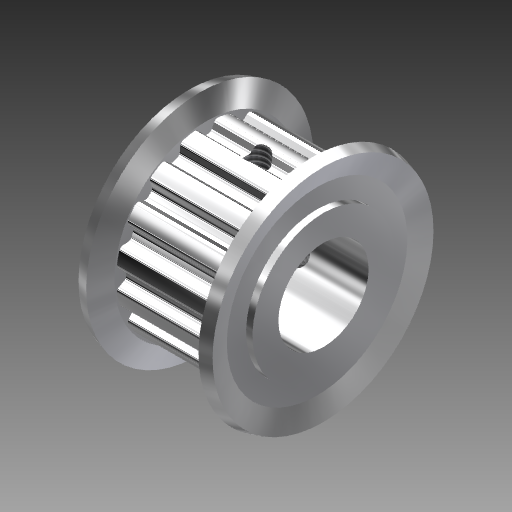
# Autodesk Inventor part: ATP16XL050-A-PUF_a
Saved by Autodesk Inventor 2019 (Build 230136000, 136)
## iProperties
Category: PARTsolutions
Company: MISUMI
Created: 2018-08-04
Part Number: ATP16XL050-A-PUF_a
Material: Aluminum 6061
Catalog Web Link: www.cadenas.de
Description: ATP_ _XL025, ATP_ _XL031, ATP_ _ XL037, ATP_ _XL050, BTP_ _XL025, BTP_ _XL031, BTP_ _XL037, BTP_ _XL050, KTP_ _XL025, KTP_ _XL031, KTP_ _ XL037, KTP_ _XL050, NTP_ _XL025, NTP_ _XL031, NTP_ _ XL037, NTP_ _XL050, MTP_ _XL025, MTP_ _ XL037, MTP_ _XL050, MTPB_ _XL025, MTPB_ _ XL037, MTPB_ _XL050, MTPP_ _XL025, MTPP_ _ XL037, MTPP_ _XL050, STP_ _XL025, STP_ _ XL037, STP_ _XL050_aI-Timing Pulleys XL Type
Vendor: MISUMI
Document SubType Name: Modeling
Designer: psadmin
Manufacturer: MISUMI
Mass: 19.1099 g
Surface Area: 46.6656 cm^2
Volume: 7.07773 cm^3
Density: 2.7 g/cm^3
Appearance: Aluminum - Flat
PSOL_IDENT_0: {$CADENAS_DATA\23d-libs\misumi\metric\51_timing_pulleys\timing_pulleys_inch\atp_xl_inch.prj},698 {VT
PSOL_IDENT_1: YP=3D},{NB=ATP16XL050-A-PUF_a},{LINA=ATP16XL050-A-PUF_a},{NN=ATP_ _XL025, ATP_ _XL031, ATP_ _ XL037,
PSOL_IDENT_2: ATP_ _XL050, BTP_ _XL025, BTP_ _XL031, BTP_ _XL037, BTP_ _XL050, KTP_ _XL025, KTP_ _XL031, KTP_ _ X
PSOL_IDENT_3: L037, KTP_ _XL050, NTP_ _XL025, NTP_ _XL031, NTP_ _ XL037, NTP_ _XL050, MTP_ _XL025, MTP_ _ XL037, M
PSOL_IDENT_4: TP_ _XL050, MTPB_ _XL025, MTPB_ _ XL037, MTPB_ _XL050, MTPP_ _XL025, MTPP_ _ XL037, MTPP_ _XL050, ST
PSOL_IDENT_5: P_ _XL025, STP_ _ XL037, STP_ _XL050_aI},{DATE=30.03.2018 07:26:26},{GEOMDATE=12.01.2011 12:59:00},{
PSOL_IDENT_6: VERSION=},{LINEID=30},{WBVAR=MATP,ST,TNW,PS,SHS,DD,ALT2,M,QSC,QFC,QTC,ALT7,K,KSC,KFC,KTC,ALT1,ALT3,A
PSOL_IDENT_7: LT4,ALT5,FC,ALT6,TPC,ALT8,BC,ALT9,SLH},{WBNUMERIC=DD,QSC,QFC,QTC,K,KSC,KFC,KTC,FC,TPC,BC,SLH}  {NB=A
PSOL_IDENT_8: TP16XL050-A-PUF_a},{LINA=ATP16XL050-A-PUF_a},{KT=DUMMY},{PN=ATP16XL050-A-PUF},{TYPE=ATP},{MATP=ATP},
PSOL_IDENT_9: {MATPA='ATP','2017 Aluminum Alloy (Duralumin)','MTP','1045 Carbon Steel','STP','304 Stainless Steel'
PSOL_IDENT_10: },{MATF=5052 Aluminum Alloy},{ST=CA},{HARD=-},{STA= 'CA' , 'Clear Anodize' , 'BA','Black Anodize','H
PSOL_IDENT_11: AT','Hard Clear Anodize','ENP' , 'Electroless Nickel Plating' },{NT=16},{TNW=XL050},{TNW1=      'XL0
PSOL_IDENT_12: 25','XL031','XL037','XL050'                            },{BW=12.7mm (1/2inch)},{A=14.0},{W=19.0},{L=
PSOL_IDENT_13: 28},{PS=A},{PSA='A','B'},{SHS=P},{SHS1= 'H','Inch Round Hole', 'P','Inch Round Hole + Tap','N','Inch
PSOL_IDENT_14: ANSI Key Groove Hole'},{SHS2=-PUF},{SHSA= 'H','Inch Round Hole', 'P','Inch Round Hole + Tap','N','I
PSOL_IDENT_15: nch ANSI Key Groove Hole'},{SHSB= 'H','Inch Round Hole', 'P','Inch Round Hole + Tap','N','Inch ANSI
PSOL_IDENT_16: Key Groove Hole'},{DD=0.5},{DDINCH=12.7},{DD1=0.25,0.3125,0.3750,0.5},{DDH=0.25,0.3125,0.3750,0.5},{
PSOL_IDENT_17: DDP=0.25,0.3125,0.3750,0.5},{DDN=0.3125,0.3750,0.5},{DDNK=10},{DDC=10,12},{DDV=5,6,6.35,7,8,9,10,11}
PSOL_IDENT_18: ,{DDF=5,6,6.35,7,8,9,10},{DDY=5,6,7,8,9,10,11,12},{DD635=13},{Z=0},{Z1=0},{ZQRMIN=15},{ZMAX=13},{ZA=
PSOL_IDENT_19: 0},{ZB=0},{ZAB=},{J=0},{JA=0},{JMAX=17.0},{JAB=},{QRMAX=14},{Q=0},{Q1=0},{Q2=},{R=0},{R1=0},{R2=},{S=
PSOL_IDENT_20: 0},{S1=0},{S2=},{SMAX=8},{T=0},{T1=0},{T2=},{TMAX=8},{PD=25.87},{OD=25.36},{D=0},{DB=17},{F=32},{E=2
PSOL_IDENT_21: 0},{DE=20},{BJS9=0},{TTTI=0},{TTT=0},{AC=-},{NDM=4.000},{WL=19},{ALT2=},{ALT2A='','N/A'},{QMIN=20},{
PSOL_IDENT_22: QMAX=13},{M=-},{MA= '-' },{MAA=},{NDMALT=0.000},{QSC=0},{QSCA=0},{QSCAA=},{QFC=0},{QFCA=0},{QFCAA=},
PSOL_IDENT_23: {QTC=0},{QTCA=0},{QTCAA=},{QCMIN=17},{QCMAX=16},{QC=0},{ALT7=},{ALT7A='','N/A'},{ALT71=1},{ALT72=1},
PSOL_IDENT_24: {ALT73=1},{K=0.0},{KSC=0},{KSCA=  [0:0]       },{KSCAA=},{KFC=0},{KFCA=  [0:0]       },{KFCAA=},{KTC=
PSOL_IDENT_25: 0},{KTCA=  [0:0]       },{KTCAA=},{KC=0},{KCMIN=17},{KCMAX=16},{KA=0},{KMAX=0.0},{KPN=},{ALT1=},{ALT
PSOL_IDENT_26: 1A='','w/o KC90 (Set Screw Angle)','-KC90','with KC90 (Set Screw Angle)'},{ALT3=},{ALT4=},{ALT4A= ''
PSOL_IDENT_27: , 'w/o Flange Attached on One Side Only', '-RFC'  , 'with RFC (Flange Attached on The hub Side Only)'
PSOL_IDENT_28: , '-LFC'  , 'with LFC (Flange Attached on The Opposite Side Only)' },{ALT5=},{ALT5A='','w/o FC (Flan
PSOL_IDENT_29: ge Cut)','-FC','with FC (Flange Cut)'},{FC=0.0},{ODAINT=25},{FCMIN=27.5},{FCMAX=30.0},{FCA=0},{FCAA=
PSOL_IDENT_30: },{ALFA=25},{ZUB=1.270},{TT=0.5},{TAP1=28.000},{TAP2=0.000},{TAP=0.000},{MM=2.5},{ALT6=},{ALT6A= '','
PSOL_IDENT_31: w/o TPC (Tapped Hole Dimension)','-TPC','with TPC (Tapped Hole Dimension)'},{TPC=0},{TPCA=
PSOL_IDENT_32: 0,'N/A'         },{TPCAA=},{ALT8=},{ALT8A=   '','N/A'                         },{BC=0.0},{BCCA=0},{
PSOL_IDENT_33: BCCAMIN=7},{BCPLANE=9.5},{BCCAMAX=9},{BCAA=},{TMP=},{KTT=6.83},{KYY=5.85},{PLANE=19},{TIF=1},{RUPE=2
PSOL_IDENT_34: },{ALT9=},{ALT9A= '','w/o SLH (Set Screw Length)','-SLH','with SLH (Set Screw Length)' },{SLH=0},{SL
PSOL_IDENT_35: HA=0},{SLHPN=},{LS=3},{WS=4},{SL=12.68},{SL2=12.68},{ANG=112.5},{SCREWALG=1},{WLBC=19},{DDPN=F},{BBI
PSOL_IDENT_36: NCH=3.125}
NN: ATP_ _XL025, ATP_ _XL031, ATP_ _ XL037, ATP_ _XL050, BTP_ _XL025, BTP_ _XL031, BTP_ _XL037, BTP_ _XL050, KTP_ _XL025, KTP_ _XL031, KTP_ _ XL037, KTP_ _XL050, NTP_ _XL025, NTP_ _XL031, NTP_ _ XL037, NTP_ _XL050, MTP_ _XL025, MTP_ _ XL037, MTP_ _XL050, MTPB_ _XL025, MTPB_ _ XL037, MTPB_ _XL050, MTPP_ _XL025, MTPP_ _ XL037, MTPP_ _XL050, STP_ _XL025, STP_ _ XL037, STP_ _XL050_aI
NT: 16
NB: ATP16XL050-A-PUF_a
NBSYN: $PN._a
LINA: ATP16XL050-A-PUF_a
PN: ATP16XL050-A-PUF
MATP: 2017 Aluminum Alloy (Duralumin)
MATF: 5052 Aluminum Alloy
ST: Clear Anodize
HARD: -
TNW: XL050
BW: 12.7mm (1/2inch)
A: 14
W: 19
L: 28
PS: A
SHS: Inch Round Hole + Tap
DD: 0
PD: 25.87
OD: 25.36
D: 0
F: 32
E: 20
AC: -
ALT2: N/A
M: -
QSC: 0
QFC: 0
QTC: 0
ALT7: N/A
K: 0
KSC: 0
KFC: 0
KTC: 0
ALT1: w/o KC90 (Set Screw Angle)
ALT3: w/o NFC (Flange not Attached)
ALT4: w/o Flange Attached on One Side Only
ALT5: w/o FC (Flange Cut)
FC: 0
ALT6: w/o TPC (Tapped Hole Dimension)
TPC: 0
ALT8: N/A
BC: 0
ALT9: w/o SLH (Set Screw Length)
SLH: 0
SUPPLIER: MISUMI
ARTICLENO: ATP16XL050-A-PUF_a
BOMINFO: ATP16XL050-A-PUF_a
CREATOR: CADENAS GmbH
Title: ATP16XL050-A-PUF_a
Author: Cadenas PARTsolutions
Comments: Timing Pulleys XL Type
Autodesk Inventor part; units mm, degrees
ref_plane "YZ Plane" through (0, 0, 0) normal (1, 0, 0) x (0, 1, 0)
ref_plane "XZ Plane" through (0, 0, 0) normal (0, 1, 0) x (-1, 0, 0)
ref_plane "XY Plane" through (0, 0, 0) normal (0, 0, 1) x (1, 0, 0)
sketch "Sketch_5" plane through (0, 0, 0) normal (0, 0, 1) x (1, 0, 0)
  line L0 (28, 0) -> (0, 0)
  line L1 (0, 6.35) -> (19, 6.35)
  line L2 (19, 6.35) -> (19, 10)
  line L3 (19, 10) -> (18.1, 10)
  line L4 (18.1, 10) -> (18.1, 12.7049)
  line L5 (18.1, 12.7049) -> (18.9352, 15.5492)
  line L6 (18.9352, 15.5492) -> (17.4, 16)
  line L7 (17.4, 16) -> (16.5, 12.935)
  line L8 (16.5, 12.935) -> (16.5, 12.68)
  line L9 (16.5, 12.68) -> (2.5, 12.68)
  line L10 (2.5, 12.68) -> (2.5, 12.935)
  line L11 (2.5, 12.935) -> (1.6, 16)
  line L12 (1.6, 16) -> (0.0648, 15.5492)
  line L13 (0.0648, 15.5492) -> (0.9, 12.7049)
  line L14 (0.9, 12.7049) -> (0.9, 10)
  line L15 (0.9, 10) -> (0, 10)
  line L16 (0, 10) -> (0, 6.35)
  constraints: 34 end point
revolve "Revolution1" add sketch "Sketch_5" angle 360 about axis through (28, 0, 0) along (1, 0, 0)
sketch "Sketch_2" plane through (2.5, 0, 0) normal (1, 0, 0) x (0, 0, -1)
  line L0 (-1.7156, 16.9067) -> (-1.7156, 12.5634)
  arc A0 (-1.0802, 12.2168) -> (-1.7156, 12.5634) centre (-1.633, 11.959) ccw
  line L1 (-1.0802, 12.2168) -> (-0.8063, 11.6295)
  arc A1 (-0.8063, 11.6295) -> (-0.2405, 11.2774) centre (-0.2535, 11.8873) ccw
  arc A2 (0.2405, 11.2774) -> (-0.2405, 11.2774) centre (0, 0) ccw
  arc A3 (0.2405, 11.2774) -> (0.8063, 11.6295) centre (0.2535, 11.8873) ccw
  line L2 (0.8063, 11.6295) -> (1.0802, 12.2168)
  arc A4 (1.7156, 12.5634) -> (1.0802, 12.2168) centre (1.633, 11.959) ccw
  line L3 (1.7156, 12.5634) -> (1.7156, 16.9067)
  line L4 (1.7156, 16.9067) -> (-1.7156, 16.9067)
  constraints: 10 end point, 10 point on circle, 5 centre point
extrude "Extrusion1" cut sketch "Sketch_2" along normal blind 14
pattern_circular "Circular Pattern1" count 16 over 360 about axis through (2.5, 0, 0) along (1, 0, 0) of "Extrusion1"
sketch "Sketch_21" plane through (9.5, 0, 0) normal (1, 0, 0) x (0, 0, -1)
  line L0 (0, 0) -> (0, 12.68)
  line L1 (0, 12.68) -> (1.621, 12.68)
  line L2 (1.621, 12.68) -> (1.621, 0)
  line L3 (1.621, 0) -> (0, 0)
  line L4 (0, 0) -> (0, 12.68)
  constraints: 10 end point
revolve "Revolution2" cut sketch "Sketch_21" angle 360 about axis through (9.5, 0, 0) along (0, -1, 0)
thread "Thread1" size "M4x0.7" class "6H" standard "ISO Metric profile" length 6.33
sketch "Sketch_22" plane through (9.5, 0, 0) normal (1, 0, 0) x (0, 0, -1)
  line L0 (0, 0) -> (11.7148, -4.8524)
  line L1 (11.7148, -4.8524) -> (11.0945, -6.35)
  line L2 (11.0945, -6.35) -> (-0.6203, -1.4976)
  line L3 (-0.6203, -1.4976) -> (0, 0)
  line L4 (0, 0) -> (11.7148, -4.8524)
  constraints: 10 end point
revolve "Revolution3" cut sketch "Sketch_22" angle 360 about axis through (9.5, 0, 0) along (0, 0.3826834, 0.9238795)
thread "Thread2" size "M4x0.7" class "6H" standard "ISO Metric profile" length 6.33
ref_plane "to_s1_XY" through (9.5, 12.68, 0) normal (0, 1, 0) x (1, 0, 0)
ref_plane "to_s1_YZ" through (9.5, 12.68, 0) normal (1, 0, 0) x (0, 0, -1)
ref_plane "to_s1_ZX" through (9.5, 12.68, 0) normal (0, 0, -1) x (0, 1, 0)
ref_plane "to_s2_XY" through (9.5, -4.8524, -11.7148) normal (0, -0.3826834, -0.9238795) x (1, 0, 0)
ref_plane "to_s2_YZ" through (9.5, -4.8524, -11.7148) normal (1, 0, 0) x (0, -0.9238795, 0.3826834)
ref_plane "to_s2_ZX" through (9.5, -4.8524, -11.7148) normal (0, -0.9238795, 0.3826834) x (0, -0.3826834, -0.9238795)
body "Solid1"
